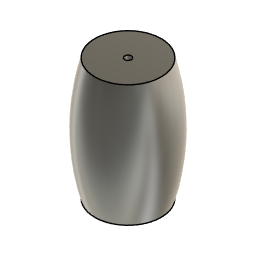
Omni_roller (Autodesk Fusion 360 design; units mm, degrees)
Autodesk Fusion 360 part; units mm, degrees
sketch "Sketch1" plane through (0, 0, 0) normal (0, 1, 0) x (1, 0, 0)
  line L0 (0.6, 0) -> (0.6, -22)
  line L1 (0.6, -22) -> (6, -22)
  line L2 (0.6, 0) -> (6, 0)
  line L3 (0.6, -11) -> (7.5, -11) construction
  arc A0 (6, -22) -> (6, 0) centre (-33.5833, -11) ccw
  dimension "d2" = 0.6
  dimension "d5" = 6.9
  dimension "d6" = 11
  dimension "d8" = 22
  dimension "d9" = 5.4
  dimension "d10" = 5.4
  constraint vertical L0
  constraint perpendicular L0 L1
  constraint perpendicular L0 L2
  constraint midpoint L0 L3.start
  constraint perpendicular L0 L3
  constraint coincident L3.end A0
  constraint coincident origin L2
  measures "d2" distance of origin L0
  measures "d5" distance of L3.start L3.end
  measures "d6" distance of L1 L3
  measures "d8" distance of L1 L2
  measures "d9" distance of L0.end L1.end
  measures "d10" distance of L0.start L2.end
revolve "Revolve1" add sketch "Sketch1" angle 360 about axis through (0, 0, 1.75) along (0, 0, 1)
equation "d5 = 7.5 mm - 0.6 mm"
equation "d6 = d8 / 2"
equation "d10 = d9"
